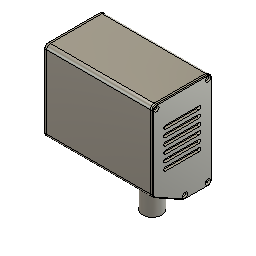
Moules_LASER v2 (Autodesk Fusion 360 design; units mm, degrees)
Autodesk Fusion 360 part; units mm, degrees
note: some values were not read from the file. Chosen so that the rebuilt part matches the saved one: a direction; which face or edge a step refers to; how an offset face is resized. Set by a fixed rule: which sketch regions a step uses.
sketch "BASE Draw" plane through (0, 0, 0) normal (1, 0, 0) x (0, 0, -1)
  line L0 (0, 0) -> (0, 80.01)
  line L1 (0, 80.01) -> (-49.01, 80.01)
  line L2 (-49.01, 80.01) -> (-49.01, 14.51)
  line L3 (-49.01, 14.51) -> (-23, 0)
  line L4 (-23, 0) -> (0, 0)
  circle A0 centre (-22.1925, 3.105) radius 1.1
  circle A1 centre (-3.105, 3.105) radius 1.1
  circle A2 centre (-45.905, 76.905) radius 1.1
  circle A3 centre (-3.105, 76.905) radius 1.1
  line L5 (-44.805, 75.805) -> (-4.205, 75.805) construction
  line L6 (-4.205, 75.805) -> (-4.205, 4.205) construction
  line L7 (-4.205, 4.205) -> (-44.805, 4.205) construction
  line L8 (-44.805, 4.205) -> (-44.805, 75.805) construction
  line L9 (-4.205, 40.005) -> (0, 40.005) construction
  line L10 (-24.505, 75.805) -> (-24.505, 80.01) construction
  circle A4 centre (-45.905, 76.905) radius 3.105
  circle A5 centre (-3.105, 76.905) radius 3.105
  circle A6 centre (-3.105, 3.105) radius 3.105
  circle A7 centre (-22.1925, 3.105) radius 3.105
  circle A8 centre (-45.905, 16.3333) radius 3.105
  dimension "d2" = 49.01
  dimension "d3" = 65.5
  dimension "d4" = 23
  dimension "d5" = 71.6
  dimension "d6" = 2.2
  dimension "d7" = 40.6
  dimension "d8" = 6.21
  dimension "d9" = 6.21
  dimension "d10" = 6.21
  dimension "d23" = 80.01
  constraint coincident L0.start L4.end
  constraint vertical L0
  constraint perpendicular L0 L1
  constraint perpendicular L1 L2
  constraint perpendicular L0 L4
  constraint horizontal L5
  constraint vertical L6
  constraint horizontal L7
  constraint vertical L8
  constraint tangent A1 L7
  constraint equal A0 A1
  constraint equal A0 A2
  constraint equal A1 A3
  constraint tangent A3 L5
  constraint midpoint L6 L9.start
  constraint midpoint L0 L9.end
  constraint horizontal L9
  constraint tangent A3 L6
  constraint tangent A1 L6
  constraint tangent A2 L8
  constraint tangent A2 L5
  constraint midpoint L5 L10.start
  constraint midpoint L1 L10.end
  constraint vertical L10
  constraint concentric A2 A4
  constraint tangent L1 A4
  constraint concentric A3 A5
  constraint tangent L1 A5
  constraint concentric A1 A6
  constraint tangent L0 A6
  constraint equal A6 A7
  constraint tangent L4 A7
  constraint tangent L3 A7
  constraint coincident A0.centre A7.centre
  constraint equal A7 A8
  constraint tangent L3 A8
  constraint tangent L2 A8
  constraint tangent L4 A6
  measures "d2" distance of L0.end L1.end
  measures "d3" distance of L1.end L2.end
  measures "d4" distance of L3.end L0.start
  measures "d5" distance of L5.end L6.end
  measures "d6" diameter of A1
  measures "d7" distance of L5.start L5.end
  measures "d8" diameter of A6
  measures "d9" diameter of A5
  measures "d10" diameter of A4
  measures "d23" distance of L0.start L0.end
sketch "Sketch1" plane through (0, 0, 0) normal (1, 0, 0) x (0, 0, -1) in component "Main_body"
extrude "Extrude1" add sketch "BASE Draw" along normal mid plane 86 contours L0 L1 L2 L3 L4 A4 A5 A6 A7 A8 | A6 | A5 | A7 | A4 | A8 makes body 1 in component "Main_body"
sketch "Sketch2" plane through (43, 0, 0) normal (1, 0, 0) x (0, 0, -1) in component "Main_body"
  circle A0 centre (-45.905, 76.905) radius 1.1
  circle A1 centre (-22.1925, 3.105) radius 1.1
  circle A2 centre (-3.105, 3.105) radius 1.1
  line L0 (-49.01, 76.905) -> (-49.01, 16.3333)
  arc A3 (-49.01, 16.3333) -> (-47.4177, 13.6217) centre (-45.905, 16.3333) ccw
  line L1 (-47.4177, 13.6217) -> (-23.7052, 0.3934)
  arc A4 (-23.7052, 0.3934) -> (-22.1925, 0) centre (-22.1925, 3.105) ccw
  line L2 (-22.1925, 0) -> (-3.105, 0)
  line L3 (0, 3.105) -> (0, 76.905)
  arc A5 (0, 76.905) -> (-3.105, 80.01) centre (-3.105, 76.905) ccw
  line L4 (-3.105, 80.01) -> (-45.905, 80.01)
  arc A6 (-45.905, 80.01) -> (-49.01, 76.905) centre (-45.905, 76.905) ccw
  line L5 (-47.01, 78.11) -> (-3, 78.11)
  line L6 (-3, 78.11) -> (-3, 1.9)
  line L7 (-3, 1.9) -> (-47.01, 1.9)
  line L8 (-47.01, 1.9) -> (-47.01, 78.11)
  line L9 (-47.01, 15.5699) -> (-22.5059, 1.9)
  circle A7 centre (-22.1925, 3.105) radius 2.05
  circle A8 centre (-3.105, 3.105) radius 2.05
  circle A9 centre (-3.105, 76.91) radius 2.05
  circle A10 centre (-45.905, 76.905) radius 2.05
  circle A11 centre (-46.01, 16.1571) radius 1
  circle A12 centre (-3.105, 76.905) radius 1.1
  arc A13 (-3.105, 0) -> (0, 3.105) centre (-3.105, 3.105) ccw
  dimension "d14" = 3
  dimension "d15" = 1.9
  dimension "d16" = 1.9
  dimension "d17" = 2
  dimension "d18" = 1.9
  dimension "d19" = 4.1
  dimension "d20" = 2
  constraint horizontal L5
  constraint vertical L6
  constraint horizontal L7
  constraint vertical L8
  constraint coincident L8 L9.start
  constraint coincident L7 L9.end
  constraint parallel L1 L9
  constraint concentric A1 A7
  constraint concentric A2 A8
  constraint concentric A0 A10
  constraint equal A7 A8
  constraint equal A8 A9
  constraint equal A9 A10
  constraint tangent L9 A11
  constraint tangent L8 A11
  measures "d14" distance of L3 L6
  measures "d15" distance of L2 L7
  measures "d16" distance of L4 L5
  measures "d17" distance of L0 L8
  measures "d18" distance of L1 L9
  measures "d19" diameter of A7
  measures "d20" diameter of A11
extrude "Extrude2" cut sketch "Sketch2" against normal through all contours L5 L6 L7 L8 L9 A7 A8 A9 A10 A11 | A11 bodies 1 in component "Main_body"
fillet "Fillet1" radius 0.5 8 edges at (0, 2.8606, 24.2279) (0, 1.9, 20.534) (0, 1.9, 4.7635) (0, 5.1523, 3) (0, 74.8627, 3) (0, 78.11, 4.7671) (0, 78.11, 44.2465) (0, 75.1783, 47.01) on bodies 1 in component "Main_body"
extrude "Extrude1'" add sketch "BASE Draw" against normal blind 2.05 from surface at -43 separate body contours L0 L1 L2 L3 L4 A4 A5 A6 A7 A8 | A6 | A5 | A7 | A4 | A8 makes body 2 in component "cap_left"
thread "Thread1" "ISO Metric profile 2.0 M2x0.4 6H" major diameter 2.074 minor diameter 1.623 pitch 0.4 angle 60 resizes the face on face at (14.3333, 2.1255, 22.6931) on face at (14.3333, 77.4911, 44.9741) on face at (14.3333, 2.2134, 3.7493) on face at (-14.3333, 76.1837, 2.2745) on bodies 1 in component "Main_body"
chamfer "Chamfer1" distance 1 angle 45 4 edges at (-45.05, 76.5072, 46.9306) (-45.05, 76.5072, 4.1306) (-45.05, 2.7072, 4.1306) (-45.05, 2.7072, 23.2181) on bodies 2 in component "cap_left"
chamfer "Chamfer1" distance 0.6 angle 45 10 edges at (-45.05, 7.0076, 35.5615) (-45.05, 14.761, 48.5825) (-45.05, 46.6192, 49.01) (-45.05, 79.1006, 48.1006) (-45.05, 80.01, 24.505) (-45.05, 79.1006, 0.9094) (-45.05, 40.005, 0) (-45.05, 0.9094, 0.9094) (-45.05, 0, 12.6487) (-45.05, 0.1, 22.974) on bodies 2 in component "cap_left"
sketch "Sketch1 (2)" plane through (-45.05, 0, 0) normal (-1, 0, 0) x (0, 0, 1) in component "cap_left"
  circle A0 centre (22.1925, 3.105) radius 2.1
  circle A1 centre (3.105, 76.905) radius 2.1
  circle A2 centre (45.905, 76.905) radius 2.1
  circle A3 centre (3.105, 3.105) radius 2.1
  line L0 (23.4129, 0.9174) -> (47.1254, 14.1457)
  arc A4 (47.1254, 14.1457) -> (48.41, 16.3333) centre (45.905, 16.3333) ccw
  line L1 (48.41, 16.3333) -> (48.41, 76.905)
  arc A5 (48.41, 76.905) -> (45.905, 79.41) centre (45.905, 76.905) ccw construction
  line L2 (45.905, 79.41) -> (3.105, 79.41) construction
  arc A6 (3.105, 79.41) -> (0.6, 76.905) centre (3.105, 76.905) ccw construction
  line L3 (0.6, 76.905) -> (0.6, 3.105)
  arc A7 (0.6, 3.105) -> (3.105, 0.6) centre (3.105, 3.105) ccw
  line L4 (3.105, 0.6) -> (22.1925, 0.6)
  arc A8 (22.1925, 0.6) -> (23.4129, 0.9174) centre (22.1925, 3.105) ccw
  line L5 (9.105, 61.51) -> (39.905, 61.51) construction
  line L6 (39.905, 61.51) -> (39.905, 28.51) construction
  line L7 (39.905, 28.51) -> (9.105, 28.51) construction
  line L8 (9.105, 28.51) -> (9.105, 61.51) construction
  line L9 (3.105, 76.905) -> (45.905, 76.905) construction
  line L10 (24.505, 76.905) -> (24.505, 33.2164) construction
  line L11 (0, 80.01) -> (49.01, 80.01) construction
  line L12 (10.605, 58.51) -> (38.405, 58.51)
  arc A9 (38.405, 58.51) -> (38.405, 61.51) centre (38.405, 60.01) ccw
  line L13 (38.405, 61.51) -> (10.605, 61.51)
  arc A10 (10.605, 61.51) -> (10.605, 58.51) centre (10.605, 60.01) ccw
  line L14 (10.605, 60.01) -> (38.405, 60.01) construction
  line L15 (38.405, 55.51) -> (10.605, 55.51)
  arc A11 (10.605, 55.51) -> (10.605, 52.51) centre (10.605, 54.01) ccw
  arc A12 (38.405, 52.51) -> (38.405, 55.51) centre (38.405, 54.01) ccw
  line L16 (10.605, 52.51) -> (38.405, 52.51)
  line L17 (38.405, 49.51) -> (10.605, 49.51)
  arc A13 (10.605, 49.51) -> (10.605, 46.51) centre (10.605, 48.01) ccw
  arc A14 (38.405, 46.51) -> (38.405, 49.51) centre (38.405, 48.01) ccw
  line L18 (10.605, 46.51) -> (38.405, 46.51)
  line L19 (38.405, 43.51) -> (10.605, 43.51)
  arc A15 (10.605, 43.51) -> (10.605, 40.51) centre (10.605, 42.01) ccw
  arc A16 (38.405, 40.51) -> (38.405, 43.51) centre (38.405, 42.01) ccw
  line L20 (10.605, 40.51) -> (38.405, 40.51)
  line L21 (38.405, 37.51) -> (10.605, 37.51)
  arc A17 (10.605, 37.51) -> (10.605, 34.51) centre (10.605, 36.01) ccw
  arc A18 (38.405, 34.51) -> (38.405, 37.51) centre (38.405, 36.01) ccw
  line L22 (10.605, 34.51) -> (38.405, 34.51)
  line L23 (38.405, 31.51) -> (10.605, 31.51)
  arc A19 (10.605, 31.51) -> (10.605, 28.51) centre (10.605, 30.01) ccw
  arc A20 (38.405, 28.51) -> (38.405, 31.51) centre (38.405, 30.01) ccw
  line L24 (10.605, 28.51) -> (38.405, 28.51)
  dimension "d29" = 33
  dimension "d30" = 30.8
  dimension "d31" = 18.5
  dimension "d32" = 3
  dimension "d36" = 0
  dimension "d37" = -30
  constraint horizontal L5
  constraint vertical L6
  constraint horizontal L7
  constraint vertical L8
  constraint coincident A1.centre A6.centre
  constraint coincident A2.centre A5.centre
  constraint midpoint L9 L10.start
  constraint perpendicular L9 L10
  constraint symmetric L6 L8 L10
  constraint tangent L12 A9
  constraint tangent A9 L13
  constraint parallel L12 L13
  constraint tangent L13 A10
  constraint tangent L12 A10
  constraint perpendicular L10 L14
  constraint tangent L8 A10
  constraint tangent L6 A9
  constraint coincident L5 A9.end
  measures "d29" distance of L5.end L6.end
  measures "d30" distance of L5.start L5.end
  measures "d31" distance of L5 L11
  measures "d32" distance of L12 L13
extrude "Extrude2'" cut sketch "Sketch1 (2)" against normal through all contours L12 A9 L13 A10 | L15 A11 A12 L16 | L17 A13 A14 L18 | L19 A15 A16 L20 | L21 A17 A18 L22 | L23 A19 A20 L24 bodies 2 in component "cap_left"
mirror "MirrorComponent1" about plane through (0, 0, 0) normal (0, 0, 1) of bodies 2 makes body 3 in component "cap_Right(Mirror)"
sketch "Sketch2 (2)" plane through (0, 0, 0) normal (0, 0, -1) x (-1, 0, 0)
  line L0 (43, 76.905) -> (-43, 76.905) construction
  line L1 (-43, 76.905) -> (-43, 3.105) construction
  line L2 (-43, 3.105) -> (43, 3.105) construction
  line L3 (43, 3.105) -> (43, 76.905) construction
  line L4 (-18.425, 65.56) -> (18.425, 65.56) construction
  line L5 (18.425, 65.56) -> (18.425, 12.91) construction
  line L6 (18.425, 12.91) -> (-18.425, 12.91) construction
  line L7 (-18.425, 12.91) -> (-18.425, 65.56) construction
  line L8 (0, 76.905) -> (0, -10.5573) construction
  circle A0 centre (-20.425, 67.56) radius 2
  circle A1 centre (20.425, 67.56) radius 2
  circle A2 centre (-20.425, 10.91) radius 2
  circle A3 centre (20.425, 10.91) radius 2
  line L9 (-29.2982, 69.56) -> (30.6617, 69.56) construction
  point P0 (43, 80.01)
  dimension "d40" = 52.65
  dimension "d42" = 36.85
  dimension "d43" = 4
  dimension "d44" = 10.45
  constraint horizontal L4
  constraint vertical L5
  constraint horizontal L6
  constraint vertical L7
  constraint midpoint L0 L8.start
  constraint perpendicular L2 L8
  constraint symmetric L5 L7 L8
  constraint equal A0 A2
  constraint equal A2 A3
  constraint equal A1 A2
  constraint tangent L4 A0
  constraint tangent L4 A1
  constraint tangent L7 A0
  constraint tangent L5 A1
  constraint tangent L6 A2
  constraint tangent L7 A2
  constraint tangent L5 A3
  constraint tangent L6 A3
  constraint perpendicular L8 L9
  constraint tangent A1 L9
  measures "d40" distance of L4.end L5.end
  measures "d42" distance of L4.start L4.end
  measures "d43" diameter of A0
  measures "d44" distance of P0 L9
extrude "Extrude3" cut sketch "Sketch2 (2)" against normal up to surface (3 mm away) bodies 1 in component "Main_body"
thread "Thread2" "ISO Metric profile 4.0 M4x0.5 6H" major diameter 4.0861 minor diameter 3.5287 pitch 0.5 angle 60 resizes the face on face at (22.1814, 68.5165, 2) on face at (-18.6686, 68.5165, 2) on face at (-22.4225, 10.8103, 2) on face at (18.4275, 10.8103, 2) on bodies 1 in component "Main_body"
sketch "LASER" plane through (0, 0, 0) normal (0, -1, 0) x (1, 0, 0)
  line L0 (-43, 3.105) -> (43, 3.105)
  line L1 (43, 3.105) -> (43, 22.1925)
  line L2 (43, 22.1925) -> (-43, 22.1925)
  line L3 (-43, 22.1925) -> (-43, 3.105)
  line L4 (28.55, 61.9103) -> (28.55, -3.4845) construction
  line L5 (45.05, 22.1925) -> (45.05, 3.105)
  circle A0 centre (18.55, 23) radius 10
  circle A1 centre (18.55, 23) radius 8
  line L6 (28.55, 15) -> (-18.4774, 15) construction
  line L7 (-43, 0) -> (43, 0)
  dimension "d47" = 16.5
  dimension "d48" = 20
  dimension "d49" = 16
  dimension "d50" = 15
  constraint perpendicular L0 L4
  constraint tangent L4 A0
  constraint concentric A0 A1
  constraint coincident L4 L6.start
  constraint perpendicular L4 L6
  constraint tangent A1 L6
  measures "d47" distance of L4 L5
  measures "d48" diameter of A0
  measures "d49" diameter of A1
  measures "d50" distance of L6 L7
extrude "Extrude4" cut sketch "LASER" against normal blind 9 contours L2 A0 A1 | L2 A0 A1 | L2 A1 | L2 A1 bodies 1 in component "Main_body"
extrude "Extrude1''" add sketch "LASER" along normal mid plane 40 separate body contours L2 A1 | L2 A1 makes body 4 in component "Laser_simple"
sketch "Sketch4" plane through (0, -20, 0) normal (0, -1, 0) x (1, 0, 0)
  circle A0 centre (18.55, 23) radius 8
  circle A1 centre (18.55, 23) radius 5.5
  dimension "d55" = 11
  constraint concentric A0 A1
  measures "d55" diameter of A1
extrude "Extrude2''" cut sketch "Sketch4" against normal blind 38 contours A1 bodies 4 in component "Laser_simple"
component "Main_body" placed x (1, 0, 0) y (0, 1, 0) z (0, 0, 1) at (0, 0, 0)
component "cap_left" placed x (1, 0, 0) y (0, 1, 0) z (0, 0, 1) at (0, 0, 0)
component "cap_Right(Mirror)" placed x (-1, 0, 0) y (0, 1, 0) z (0, 0, -1) at (0, 0, 0)
component "Laser_simple" placed x (1, 0, 0) y (0, 1, 0) z (0, 0, 1) at (0, 0, 0)
equation "d11 = Main_body_size"
equation "Main_body_size = 86 mm"
equation "d18 = d15"
equation "d29 = Spacing_grid_LEFTCAP"
equation "Spacing_grid_LEFTCAP = 33 mm"
equation "d37 = -Spacing_grid_LEFTCAP + 3 mm"
